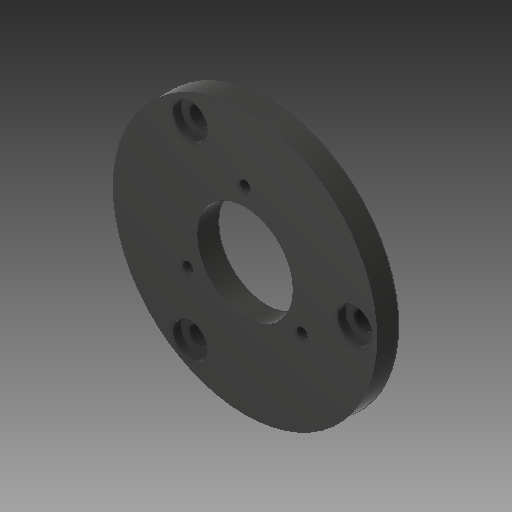
# Autodesk Inventor part: Encoder Mount Front
Saved by Autodesk Inventor 2018 (Build 220112000, 112)
## iProperties
Created: 2018-03-20
Part Number: Encoder Mount Front
Material: ABS Plastic
Document SubType Name: Modeling
Designer: P301319
Density: 1.06 g/cm^3
Appearance: Smooth - Black
Mass: 12.4212 g
Surface Area: 64.5362 cm^2
Volume: 11.7181 cm^3
Author: P301319
Autodesk Inventor part; units mm, degrees
ref_plane "YZ Plane" through (0, 0, 0) normal (1, 0, 0) x (0, 1, 0)
ref_plane "XZ Plane" through (0, 0, 0) normal (0, 1, 0) x (-1, 0, 0)
ref_plane "XY Plane" through (0, 0, 0) normal (0, 0, 1) x (1, 0, 0)
sketch "Sketch1" plane through (0, 0, 0) normal (0, 0, 1) x (1, 0, 0)
  circle A0 centre (0, 0) radius 10
  circle A1 centre (0, 0) radius 30
  circle A2 centre (0, 15) radius 1.25
  circle A3 centre (-12.9904, -7.5) radius 1.25
  circle A4 centre (12.9904, -7.5) radius 1.25
  dimension "d0" = 20
  dimension "d1" = 60
  dimension "d3" = 2.5
  dimension "d6" = 360
  constraints: 5 centre point, 2 coincident, 7 other
  measures "d0" diameter of A0
  measures "d1" diameter of A1
  measures "d3" diameter of A2
extrude "Extrusion1" add sketch "Sketch1" along normal blind 5
sketch "Sketch5" plane through (0, 0, 5) normal (0, 0, 1) x (1, 0, 0)
  circle A0 centre (0, 0) radius 25 construction
  circle A1 centre (25, 0) radius 2.25
  dimension "d40" = 50
  dimension "d41" = 4.5
  constraints: 2 horizontal alignment, 1 centre point, 1 coincident, 2 other
  measures "d41" diameter of A1
hole "Hole1" at (25, 0, 5) direction (0, 0, -1) diameter 4.5 end through all counterbore diameter 8 counterbore depth 2
pattern_circular "Circular Pattern2" count 3 over 360 about axis through (0, 0, 0) along (0, 0, 1) of "Hole1"
sketch "Sketch4" plane through (0, 0, 5) normal (0, 0, 1) x (1, 0, 0)
  circle A0 centre (0, 0) radius 10 projected
  circle A1 centre (0, 0) radius 11
  dimension "d34" = 1
  constraints: 1 centre point
  measures "d34" radial gap between concentric circles of A0 A1
extrude "Extrusion8" cut sketch "Sketch4" against normal blind 10
body "Solid1"
